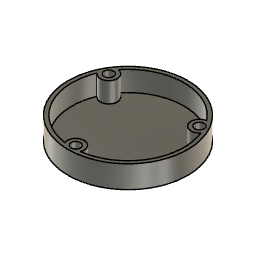
Base module generator (Autodesk Fusion 360 design; units mm, degrees)
Autodesk Fusion 360 part; units mm, degrees
sketch "Schizzo1" plane through (0, 0, 0) normal (0, 0, 1) x (1, 0, 0)
  circle A0 centre (-60.6218, 35) radius 6.1
  line L0 (-60.6218, 35) -> (0, -70) construction
  line L1 (0, -70) -> (60.6218, 35) construction
  circle A1 centre (0, -70) radius 6.1
  circle A2 centre (60.6218, 35) radius 6.3
  circle A3 centre (-60.6218, 35) radius 6.3
  circle A4 centre (0, 0) radius 80
  line L2 (60.6218, 35) -> (-60.6218, 35) construction
  circle A5 centre (0, 0) radius 70 construction
  circle A6 centre (60.6218, 35) radius 6.1
  circle A7 centre (0, -70) radius 6.3
  line L3 (0, 0) -> (0, -70) construction
  dimension "d1" = 140
  dimension "d2" = 10
  dimension "d3" = 0.2
  dimension "d4" = 12.2
  constraint coincident A4.centre A5.centre
  constraint coincident L0.end A5
  constraint vertical L3
  constraint coincident L0.end L1.start
  constraint coincident L1.end A5
  constraint coincident A0.centre A5
  constraint horizontal L2
  constraint equal L1 L2
  constraint coincident L1.end A2.centre
  constraint coincident A0.centre L0.start
  constraint equal A3 A7
  constraint equal A2 A7
  constraint concentric A0 A3
  constraint concentric A1 A7
  constraint concentric A2 A6
  constraint equal A1 A6
  constraint equal A0 A1
  measures "d1" diameter of A5
  measures "d2" distance of A4 A5
  measures "d3" distance of A1 A7
  measures "d4" diameter of A1
extrude "Estrusione2" add sketch "Schizzo1" along normal blind 27 contours A4
shell "Svuotamento1" thickness 5 removed faces 2 at (-0.1569, -0.2718, 27) at (-0.1569, -0.2718, 0)
extrude "Estrusione1" add sketch "Schizzo1" against normal blind 3 contours A4
equation "Floor_Thickness = 3 mm"
equation "Wall_Thickness = 5 mm"
equation "Height = 30 mm" comment "Will include Floor_Thickness"
equation "d8 = -Floor_Thickness"
equation "d10 = Height - Floor_Thickness"
equation "d12 = Wall_Thickness"
equation "Roof_Thickness = 0 mm"
